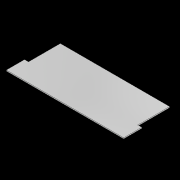
# Autodesk Inventor part: TopBottomPlates
Saved by Autodesk Inventor 2021 (Build 250183000, 183)
## iProperties
Created: 2021-03-10
Part Number: TopBottomPlates
Material: Aluminum 6061
Document SubType Name: Modeling
Designer: Dylan
Density: 2.7 g/cm^3
Appearance: Aluminum - Polished
Mass: 7184.28 g
Surface Area: 7116.28 cm^2
Volume: 2660.84 cm^3
Author: Dylan
Autodesk Inventor part; units mm, degrees
ref_plane "YZ Plane" through (0, 0, 0) normal (1, 0, 0) x (0, 1, 0)
ref_plane "XZ Plane" through (0, 0, 0) normal (0, 1, 0) x (-1, 0, 0)
ref_plane "XY Plane" through (0, 0, 0) normal (0, 0, 1) x (1, 0, 0)
sketch "Sketch1" plane through (0, 0, 0) normal (0, 1, 0) x (-1, 0, 0)
  line L0 (0, 0) -> (780.8383, 0)
  line L1 (780.8383, 0) -> (780.8383, -332.74)
  line L2 (780.8383, -332.74) -> (0, -332.74)
  line L3 (0, -332.74) -> (0, 0)
  line L4 (780.8383, -332.74) -> (754.2742, -332.74)
  line L5 (754.2742, -332.74) -> (754.2742, -120.65)
  line L6 (754.2742, -120.65) -> (780.8383, -120.65)
  line L7 (780.8383, -120.65) -> (780.8383, -332.74)
  line L8 (0, -332.74) -> (26.5642, -332.74)
  line L9 (26.5642, -332.74) -> (26.5642, -120.65)
  line L10 (26.5642, -120.65) -> (0, -120.65)
  line L11 (0, -120.65) -> (0, -332.74)
  dimension "d0" = 780.8383
  dimension "d1" = 332.74
  dimension "d3" = 120.65
  dimension "d4" = 26.5642
  constraints: 24 end point, 6 parallel, 3 horizontal, 3 perpendicular, 1 collinear, 1 point on line
  measures "d0" distance of L1.end L2.end
  measures "d1" distance of L0.end L1.end
  measures "d3" distance between parallel lines of L0 L6
  measures "d4" distance of L5.end L6.end
extrude "Extrusion1" add sketch "Sketch1" along normal blind 6.35 contours L0 L1 L6 L5 L2 L9 L10 L3
body "Solid1"
